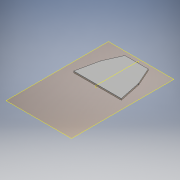
# Autodesk Inventor part: tværplade
Saved by Autodesk Inventor 2018 (Build 220112000, 112)
## iProperties
Created: 2019-09-28
Part Number: tværplade
Material: S355MC
Document SubType Name: Sheet Metal
Designer: loppen
Density: 7.85 g/cm^3
Sheet Metal Rule: Default_mm
Appearance: Light Gray
Mass: 131.54 g
Surface Area: 120.658 cm^2
Volume: 16.7567 cm^3
Author: loppen
Autodesk Inventor part; units mm, degrees
ref_plane "YZ Plane" through (0, 0, 0) normal (1, 0, 0) x (0, 1, 0)
ref_plane "XZ Plane" through (0, 0, 0) normal (0, 1, 0) x (-1, 0, 0)
ref_plane "XY Plane" through (0, 0, 0) normal (0, 0, 1) x (1, 0, 0)
ref_plane "Work Plane1" through (16.5341, 952.9567, 0) normal (0, 0, 1) x (-1, 0, 0)
sketch "Sketch1" plane through (16.5341, 952.9567, 0) normal (0, 0, 1) x (-1, 0, 0)
  line L0 (60, 40.2719) -> (60, 137.1193)
  ellipse E0 centre (56, 137.1193) end of major axis (56, 141.9614) minor radius 4 (60, 137.1193) -> (56, 141.9614) ccw
  line L1 (56, 141.9614) -> (24.75, 141.9614)
  line L2 (24.75, 141.9614) -> (24.75, 144.3824)
  line L3 (24.75, 144.3824) -> (24.75, 146.8034)
  line L4 (24.75, 146.8034) -> (56, 146.8034)
  ellipse E1 centre (56, 137.1193) end of major axis (56, 146.8034) minor radius 8 (64, 137.1193) -> (56, 146.8034) ccw
  line L5 (64, 137.1193) -> (64, 40.2719)
  ellipse E2 centre (56, 40.2719) end of major axis (56, 30.5879) minor radius 8 (63.7591, 37.9134) -> (64, 40.2719) ccw
  line L6 (63.7591, 37.9134) -> (43.4204, -60.1335)
  ellipse E3 centre (35.6613, -57.775) end of major axis (35.6613, -67.459) minor radius 8 (42.7123, -62.3499) -> (43.4204, -60.1335) ccw
  line L7 (42.7123, -62.3499) -> (7.051, -142.8866)
  ellipse E4 centre (0, -138.3116) end of major axis (0, -147.9957) minor radius 8 (-7.051, -142.8866) -> (7.051, -142.8866) ccw
  line L8 (-7.051, -142.8866) -> (-42.7123, -62.3499)
  ellipse E5 centre (-35.6613, -57.775) end of major axis (-35.6613, -67.459) minor radius 8 (-43.4204, -60.1335) -> (-42.7123, -62.3499) ccw
  line L9 (-43.4204, -60.1335) -> (-63.7591, 37.9134)
  ellipse E6 centre (-56, 40.2719) end of major axis (-56, 30.5879) minor radius 8 (-64, 40.2719) -> (-63.7591, 37.9134) ccw
  line L10 (-64, 40.2719) -> (-64, 137.1193)
  ellipse E7 centre (-56, 137.1193) end of major axis (-56, 146.8034) minor radius 8 (-56, 146.8034) -> (-64, 137.1193) ccw
  line L11 (-56, 146.8034) -> (-24.75, 146.8034)
  line L12 (-24.75, 146.8034) -> (-24.75, 144.3824)
  line L13 (-24.75, 144.3824) -> (-24.75, 141.9614)
  line L14 (-24.75, 141.9614) -> (-56, 141.9614)
  ellipse E8 centre (-56, 137.1193) end of major axis (-56, 141.9614) minor radius 4 (-56, 141.9614) -> (-60, 137.1193) ccw
  line L15 (-60, 137.1193) -> (-60, 40.2719)
  ellipse E9 centre (-56, 40.2719) end of major axis (-56, 35.4299) minor radius 4 (-60, 40.2719) -> (-59.8796, 39.0927) ccw
  line L16 (-59.8796, 39.0927) -> (-39.5409, -58.9542)
  ellipse E10 centre (-35.6613, -57.775) end of major axis (-35.6613, -62.617) minor radius 4 (-39.5409, -58.9542) -> (-39.1868, -60.0624) ccw
  line L17 (-39.1868, -60.0624) -> (-3.5255, -140.5991)
  ellipse E11 centre (0, -138.3116) end of major axis (0, -143.1536) minor radius 4 (-3.5255, -140.5991) -> (3.5255, -140.5991) ccw
  line L18 (3.5255, -140.5991) -> (39.1868, -60.0624)
  ellipse E12 centre (35.6613, -57.775) end of major axis (35.6613, -62.617) minor radius 4 (39.1868, -60.0624) -> (39.5409, -58.9542) ccw
  line L19 (39.5409, -58.9542) -> (59.8796, 39.0927)
  ellipse E13 centre (56, 40.2719) end of major axis (56, 35.4299) minor radius 4 (59.8796, 39.0927) -> (60, 40.2719) ccw
  line L20 (-24.75, 141.9614) -> (24.75, 141.9614)
  line L21 (-24.0389, -94.2722) -> (24.0389, -94.2722)
  line L22 (-48.8096, -14.2722) -> (48.8096, -14.2722)
  point P0 (16.5341, 952.9567)
  point P1 (60, -19.5271)
  dimension "d3" = 88.0788
  dimension "d4" = 44.0394
  dimension "d12" = 80
  constraints: 46 end point, 8 vertical, 5 horizontal, 4 point on line, 2 parallel, 112 other
  measures "d3" distance of L18.start L18.end
  measures "d4" distance from line of point (0, -138.312) L21
  measures "d12" distance between parallel lines of L22 L21
extrude "Plate1" add sketch "Sketch1" along normal blind 3 contours L19 E12 L18 L21 L17 E10 L16 L22
ref_plane "modplan parallel med plade" through (16.5341, 952.9567, 1.5) normal (0, 0, 1) x (1, 0, 0)
sketch "Sketch3" plane through (16.5341, 952.9567, 0) normal (0, 0, -1) x (-1, 0, 0)
  ellipse E0 centre (-35.6613, 57.775) end of major axis (-35.6613, 62.617) minor radius 4 (-39.1868, 60.0624) -> (-39.5409, 58.9542) ccw projected
  line L0 (-48.8096, 14.2722) -> (-39.5409, 58.9542) projected
  line L1 (48.8096, 14.2722) -> (-48.8096, 14.2722) projected
  line L2 (39.5409, 58.9542) -> (48.8096, 14.2722) projected
  ellipse E1 centre (35.6613, 57.775) end of major axis (35.6613, 62.617) minor radius 4 (39.5409, 58.9542) -> (39.1868, 60.0624) ccw projected
  line L3 (24.0389, 94.2722) -> (39.1868, 60.0624) projected
  line L4 (-24.0389, 94.2722) -> (24.0389, 94.2722) projected
  line L5 (-39.1868, 60.0624) -> (-24.0389, 94.2722) projected
  line L6 (-37.3581, 59.2527) -> (-22.7372, 92.2722)
  line L7 (-22.7372, 92.2722) -> (22.7372, 92.2722)
  line L8 (22.7372, 92.2722) -> (37.3581, 59.2527)
  line L9 (37.5826, 58.548) -> (46.3522, 16.2722)
  line L10 (46.3522, 16.2722) -> (-46.3522, 16.2722)
  line L11 (-46.3522, 16.2722) -> (-37.5826, 58.548)
  spline S0 degree 3 poles (-37.5826, 58.548) (-37.5324, 58.7898) (-37.4581, 59.0268) (-37.3581, 59.2527) knots 0 0 0 0 1 1 1 1
  spline S1 degree 3 poles (37.3581, 59.2527) (37.4581, 59.0268) (37.5324, 58.7898) (37.5826, 58.548) knots 0 0 0 0 1 1 1 1
  point P0 (16.5341, -952.9567)
  dimension "d14" = 2
  constraints: 12 end point, 3 parallel, 12 other
  measures "d14" distance between parallel lines of L0 L11
extrude "2 mm mindre" cut sketch "Sketch3" against normal blind 3
ref_plane "midtplan" through (16.5341, 1192.6796, 0) normal (-1, 0, 0) x (0, 0, 1)
equation "\"d4\" = 0.5 * d3"
equation "\"d15\" = Thickness"
equation "\"d8\" = Thickness"
equation "\"BendRadius\" = Thickness"
equation "\"BendReliefWidth\" = Thickness"
equation "\"BendReliefDepth\" = 0.5 * Thickness"
equation "\"CornerReliefSize\" = 4 * Thickness"
equation "\"MinimumRemnant\" = 2 * Thickness"
equation "\"TransitionRadius\" = BendRadius"
equation "\"JacobiRadiusSize\" = BendRadius"
equation "\"GapSize\" = Thickness"
equation "\"Thickness\" = 3"
body "Solid1"
